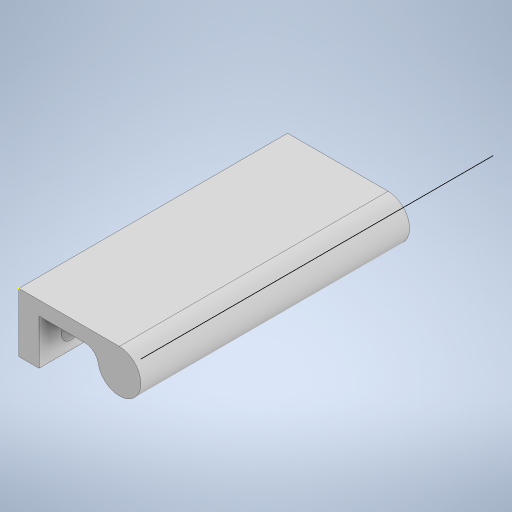
# Autodesk Inventor part: knuckle plate
Saved by Autodesk Inventor 2024.2 (Build 282272000, 272)
## iProperties
Created: 2024-08-26
Part Number: knuckle plate
Material: Generic
Document SubType Name: Modeling
Designer: Tom
Density: 1 g/cm^3
Appearance: Default
Author: Tom
Autodesk Inventor part; units mm, degrees
ref_plane "YZ Plane" through (0, 0, 0) normal (1, 0, 0) x (0, 1, 0)
ref_plane "XZ Plane" through (0, 0, 0) normal (0, 1, 0) x (-1, 0, 0)
ref_plane "XY Plane" through (0, 0, 0) normal (0, 0, 1) x (1, 0, 0)
sketch "Sketch1" plane through (0, 0, 0) normal (1, 0, 0) x (0, 1, 0)
  line L0 (0, 0) -> (13.97, 0)
  line L1 (13.97, 0) -> (13.97, -63.5)
  line L2 (13.97, -63.5) -> (0, -63.5)
  line L3 (0, -63.5) -> (0, 0)
  circle A0 centre (4.445, -7.62) radius 2.4329
  circle A1 centre (4.445, -15.6185) radius 2.4329
  circle A2 centre (4.445, -23.6169) radius 2.4329
  circle A3 centre (4.445, -31.6154) radius 2.4329
  circle A4 centre (4.445, -39.6138) radius 2.4329
  circle A5 centre (4.445, -47.6123) radius 2.4329
  circle A6 centre (4.445, -55.6108) radius 2.4329
  dimension "d0" = 63.5
  dimension "d1" = 13.97
  dimension "d3" = 9.525
  dimension "d6" = 7.9985
  dimension "d11" = 7.62
  constraints: 8 end point, 7 centre point, 2 parallel, 1 horizontal, 1 perpendicular, 1 vertical, 12 other
  measures "d0" distance of L0.end L1.end
  measures "d1" distance of L0.start L0.end
  measures "d3" distance from line of L1 A0.centre
  measures "d6" distance of A0.centre A1.centre
  measures "d11" distance from line of L0 A0.centre
extrude "Extrusion1" add sketch "Sketch1" along normal blind 4.7625
sketch "Sketch2" plane through (4.7625, 0, 0) normal (1, 0, 0) x (0, 0, -1)
  line L0 (63.5, 13.97) -> (0, 13.97) projected
  line L1 (63.5, 0) -> (63.5, 13.97) projected
  line L2 (0, 13.97) -> (63.5, 13.97)
  line L3 (63.5, 13.97) -> (63.5, 10.668)
  line L4 (63.5, 10.668) -> (0, 10.668)
  line L5 (0, 10.668) -> (0, 13.97)
  point P0 (0, 0)
  dimension "d14" = 3.302
  constraints: 8 end point, 2 parallel, 1 horizontal, 1 perpendicular, 1 point on line
  measures "d14" distance between parallel lines of L4 L0
extrude "Extrusion2" add sketch "Sketch2" along normal blind 1.016
sketch "Sketch3" plane through (0, 0, 0) normal (0, 0, 1) x (1, 0, 0)
  line L0 (5.7785, 13.97) -> (5.7785, 10.668) projected
  arc A0 (18.7423, 8.0303) -> (23.749, 13.97) centre (23.749, 8.89) ccw
  line L1 (0, 13.97) -> (0, 0) projected
  line L2 (5.7785, 13.97) -> (23.749, 13.97)
  line L3 (4.7625, 10.668) -> (5.7785, 10.668) projected
  line L4 (5.7785, 10.668) -> (15.6131, 10.668)
  arc A1 (18.7423, 8.0303) -> (15.6131, 10.668) centre (15.6131, 7.493) ccw
  point P0 (18.9903, 10.668)
  point P1 (9.5258, 13.208)
  dimension "d17" = 23.749
  dimension "d18" = 10.16
  dimension "d19" = 3.175
  constraints: 5 point on circle, 4 end point, 3 tangent, 2 centre point, 1 collinear, 1 horizontal, 1 point on line
  measures "d17" distance from line of L1 A0.centre
  measures "d18" diameter of A0
  measures "d19" radius of A1
extrude "Extrusion3" add sketch "Sketch3" against normal blind 63.5
sketch "Sketch4" plane through (0, 13.97, 0) normal (0, 1, 0) x (1, 0, 0)
  line L0 (28.829, 0) -> (28.829, 63.5) projected
  line L1 (28.829, 0) -> (28.829, 83.2403)
  point P0 (0, 0)
  constraints: 2 end point, 1 point on line, 1 vertical
body "Solid1"
